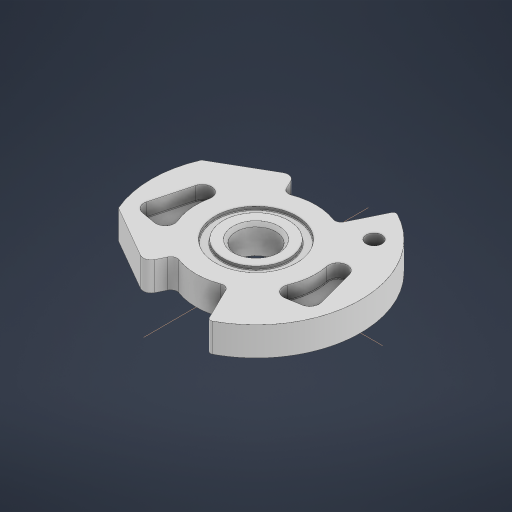
# Autodesk Inventor part: Part2
Saved by Autodesk Inventor 2023 (Build 270158000, 158)
## iProperties
Created: 2022-11-23
Part Number: Part2
Material: Generic
Document SubType Name: Modeling
Designer: iusti
Density: 1 g/cm^3
Appearance: Default
Author: iusti
Autodesk Inventor part; units mm, degrees
ref_plane "YZ Plane" through (0, 0, 0) normal (1, 0, 0) x (0, 1, 0)
ref_plane "XZ Plane" through (0, 0, 0) normal (0, 1, 0) x (-1, 0, 0)
sketch "Sketch4" plane through (0, 0, 0) normal (0, 1, 0) x (-1, 0, 0)
  arc A0 (0, 33.2) -> (-14.553922, 29.839962) centre (0, 0) ccw construction
  arc A1 (0, 19) -> (-6.664803, 17.792706) centre (0, 0) ccw
  line L0 (9.163949, 18.788881) -> (10.530343, 21.590403)
  line L1 (14.027328, 22.659539) -> (30.480188, 13.160476)
  line L2 (-9.163949, 18.788881) -> (-14.108742, 28.927208)
  line L3 (0, -52.865592) -> (0, 52.865592) construction
  line L4 (46.814748, 0) -> (-46.535791, 0) construction
  arc A2 (30.480188, 13.160476) -> (0, 33.2) centre (0, 0) ccw construction
  arc A3 (-15.473609, 29.373584) -> (-15.473609, -29.373584) centre (0, 0) ccw
  arc A4 (6.664803, 17.792706) -> (0, 19) centre (0, 0) ccw
  arc A5 (-6.664803, -17.792706) -> (8.329052, -17.077087) centre (0, 0) ccw
  arc A6 (-14.553922, -29.839962) -> (0, -33.2) centre (0, 0) ccw construction
  arc A7 (-8.329052, -17.077087) -> (0, -19) centre (0, 0) ccw construction
  line L5 (9.163949, -18.788881) -> (10.530343, -21.590403)
  line L6 (14.027328, -22.659539) -> (30.480188, -13.160476)
  line L7 (-9.163949, -18.788881) -> (-14.108742, -28.927208)
  arc A8 (0, -33.2) -> (30.480188, -13.160476) centre (0, 0) ccw construction
  arc A9 (0, -19) -> (6.664803, -17.792706) centre (0, 0) ccw construction
  arc A10 (-14.553922, -29.839962) -> (0, -33.2) centre (0, 0) ccw construction
  arc A11 (30.480188, -13.160476) -> (30.480188, 13.160476) centre (0, 0) ccw
  arc A12 (6.664803, 17.792706) -> (9.163949, 18.788881) centre (7.366361, 19.665623) ccw
  arc A13 (-9.163949, 18.788881) -> (-6.664803, 17.792706) centre (-7.366361, 19.665623) ccw
  arc A14 (9.163949, -18.788881) -> (6.664803, -17.792706) centre (7.366361, -19.665623) ccw
  arc A15 (-6.664803, -17.792706) -> (-9.163949, -18.788881) centre (-7.366361, -19.665623) ccw
  arc A16 (14.027328, 22.659539) -> (10.530343, 21.590403) centre (12.777328, 20.494476) ccw
  arc A17 (10.530343, -21.590403) -> (14.027328, -22.659539) centre (12.777328, -20.494476) ccw
  arc A18 (-14.108742, 28.927208) -> (-15.473609, 29.373584) centre (-15.007536, 28.488837) ccw
  arc A19 (-15.473609, -29.373584) -> (-14.108742, -28.927208) centre (-15.007536, -28.488837) ccw
  circle A20 centre (0, 0) radius 6.3
  point P0 (8.329052, 17.077087)
  point P1 (11.705582, 24)
  point P2 (-8.329052, 17.077087)
  point P3 (11.705582, -24)
  point P4 (6.664803, -17.792706)
  dimension "d21" = 66.4
  dimension "d23" = 26
  dimension "d24" = 52
  dimension "d25" = 30
  dimension "d26" = 48
  dimension "d27" = 19
  dimension "d30" = 2
  dimension "d31" = 2.5
  dimension "d32" = 1
  dimension "d33" = 12.6
  constraints: 46 point on circle, 21 centre point, 16 point on line, 16 tangent, 12 end point, 7 symmetric about line, 5 coincident, 5 equal radius, 4 other
  measures "d21" diameter of A0
  measures "d23" angle of L3 L2
  measures "d24" angle of L2 L0
  measures "d25" angle of L4 L1
  measures "d26" distance of point (11.706, -24) point (11.706, 24)
  measures "d27" radius of A4
  measures "d30" radius of A12
  measures "d31" radius of A16
  measures "d32" radius of A18
  measures "d33" diameter of A20
extrude "Extrusion2" add sketch "Sketch4" along normal blind 9.1
sketch "Sketch5" plane through (0, 9.1, 0) normal (0, 1, 0) x (1, 0, 0)
  arc A0 (-17.508044, -7.380271) -> (-18.606466, 3.847002) centre (0, 0) ccw construction
  line L0 (-46.48, 0) -> (46.48, 0) construction
  arc A1 (-20.793416, -11.5) -> (-17.508044, -7.380271) centre (-20.272472, -8.545577) ccw
  arc A2 (-18.606466, 3.847002) -> (-24.442107, 5.23088) centre (-21.544329, 4.454423) ccw
  line L1 (-20.793416, -11.5) -> (-25.334082, -10.699358)
  line L2 (-27.710915, -6.968478) -> (-24.442107, 5.23088)
  arc A3 (-27.710915, -6.968478) -> (-25.334082, -10.699358) centre (-24.813137, -7.744935) ccw
  line L3 (0, 41.284372) -> (0, -41.284372) construction
  arc A4 (-19, 0) -> (-17.508044, -7.380271) centre (0, 0) ccw
  arc A5 (-18.606466, 3.847002) -> (-19, 0) centre (0, 0) ccw
  arc A6 (17.508044, -7.380271) -> (20.793416, -11.5) centre (20.272472, -8.545577) ccw
  arc A7 (24.442107, 5.23088) -> (18.606466, 3.847002) centre (21.544329, 4.454423) ccw
  line L4 (20.793416, -11.5) -> (25.334082, -10.699358)
  line L5 (27.710915, -6.968478) -> (24.442107, 5.23088)
  arc A8 (25.334082, -10.699358) -> (27.710915, -6.968478) centre (24.813137, -7.744935) ccw
  arc A9 (17.508044, -7.380271) -> (19, 0) centre (0, 0) ccw
  arc A10 (19, 0) -> (18.606466, 3.847002) centre (0, 0) ccw
  dimension "d34" = 38
  dimension "d38" = 6
  dimension "d39" = 6
  dimension "d40" = 3
  dimension "d41" = 10
  dimension "d42" = 13
  dimension "d43" = 11.5
  dimension "d44" = 15
  constraints: 22 point on circle, 11 centre point, 10 symmetric about line, 8 end point, 6 tangent, 1 coincident, 1 point on line, 5 other
  measures "d34" diameter of A0
  measures "d38" diameter of A1
  measures "d39" diameter of A2
  measures "d40" radius of A3
  measures "d41" angle of L0 L1
  measures "d42" vertical distance of A2.centre A1.centre
  measures "d43" distance from line of L0 L1.start
  measures "d44" angle of L3 L2
extrude "Extrusion3" cut sketch "Sketch5" against normal blind 4.3
fillet "Fillet1" radius 0.2 12 edges at (-20.8521, 4.8, -7.3735) (-18.9097, 4.8, 1.85) (-17.927, 4.8, 10.416) (-23.0637, 4.8, 11.0997) (-27.3433, 4.8, 9.3568) (-26.0765, 4.8, 0.8688) (20.8521, 4.8, -7.3735) (26.0765, 4.8, 0.8688) (27.3433, 4.8, 9.3568) (23.0637, 4.8, 11.0997) (17.927, 4.8, 10.416) (18.9097, 4.8, 1.85)
sketch "Sketch6" plane through (0, 9.1, 0) normal (0, 1, 0) x (1, 0, 0)
  circle A0 centre (0, 0) radius 10.4
  circle A1 centre (0, 0) radius 12.9
  dimension "d48" = 20.8
  dimension "d49" = 25.8
  constraints: 2 centre point, 2 coincident
  measures "d48" diameter of A0
  measures "d49" diameter of A1
extrude "Extrusion4" cut sketch "Sketch6" against normal blind 1
fillet "Fillet2" radius 0.2 2 edges at (-10.4, 8.1, 0) (-12.9, 8.1, 0)
ref_plane "Work Plane1" through (0, 0.7, 0) normal (0, -1, 0) x (1, 0, 0)
sketch "Sketch7" plane through (0, 0.7, 0) normal (0, -1, 0) x (1, 0, 0)
  line L0 (26.595086, 11) -> (-26.595086, -11) construction
  line L1 (-26.595086, 11) -> (26.595086, -11) construction
  arc A0 (-22.782725, 10.886228) -> (-22.782725, -10.886228) centre (0, 0) ccw
  arc A1 (22.782725, -10.886228) -> (22.782725, 10.886228) centre (0, 0) ccw
  arc A2 (-17.488654, 10.695652) -> (-17.488654, -10.695652) centre (0, 0) ccw
  arc A3 (17.488654, -10.695652) -> (17.488654, 10.695652) centre (0, 0) ccw
  line L2 (-22.602268, -11) -> (-17.659275, -11)
  line L3 (17.659275, -11) -> (22.602268, -11)
  line L4 (22.602268, 11) -> (17.659275, 11)
  line L5 (-17.659275, 11) -> (-22.602268, 11)
  arc A4 (-17.659275, -11) -> (-17.488654, -10.695652) centre (-17.659275, -10.8) ccw
  arc A5 (-22.782725, -10.886228) -> (-22.602268, -11) centre (-22.602268, -10.8) ccw
  arc A6 (-22.602268, 11) -> (-22.782725, 10.886228) centre (-22.602268, 10.8) ccw
  arc A7 (-17.488654, 10.695652) -> (-17.659275, 11) centre (-17.659275, 10.8) ccw
  arc A8 (17.659275, 11) -> (17.488654, 10.695652) centre (17.659275, 10.8) ccw
  arc A9 (22.782725, 10.886228) -> (22.602268, 11) centre (22.602268, 10.8) ccw
  arc A10 (22.602268, -11) -> (22.782725, -10.886228) centre (22.602268, -10.8) ccw
  arc A11 (17.488654, -10.695652) -> (17.659275, -11) centre (17.659275, -10.8) ccw
  point P0 (-22.728011, -11)
  point P1 (-22.728011, 11)
  point P2 (17.298844, 11)
  point P3 (-17.298844, 11)
  point P4 (22.728011, 11)
  point P5 (22.728011, -11)
  point P6 (-17.298844, -11)
  point P7 (17.298844, -11)
  dimension "d58" = 0.2
  constraints: 32 point on circle, 16 tangent, 12 centre point, 12 end point, 8 point on line, 7 equal radius, 4 parallel, 2 coincident, 2 horizontal, 2 midpoint
  measures "d58" radius of A4
extrude "Extrusion5" cut sketch "Sketch7" along normal through all draft 60
chamfer "Chamfer1" distance 1 angle 45 1 edges at (6.3, 9.1, 0)
chamfer "Chamfer2" distance 0.2 angle 45 1 edges at (6.3, 0, 0)
sketch "Sketch8" plane through (0, 9.1, 0) normal (0, 1, 0) x (1, 0, 0)
  line L0 (0, 0) -> (18.73833, 18.73833) construction
  line L1 (0, 41.284372) -> (0, -41.284372)
  dimension "d67" = 45
  dimension "d68" = 26.5
  constraints: 2 end point
  measures "d67" angle of L1 L0
  measures "d68" distance of L0.end L0.start
hole "Hole2" at (18.73833, 9.1, -18.73833) direction (0, -1, 0) diameter 5 end through all
body "Solid2"
